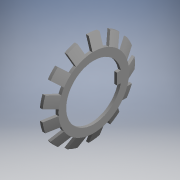
# Autodesk Inventor part: SKF_MB 5
Saved by Autodesk Inventor 2017.3 (Build 213256000, 256)
## iProperties
Part Number: SKF_MB 5
Material: Generic
Catalog Web Link: www.cadenas.de
Description: ANL_002-MB(L) lock washers
Vendor: SKF
Document SubType Name: Modeling
Designer: partserver
Manufacturer: SKF
Mass: 6 g
Surface Area: 17.574 cm^2
Volume: 0.811214 cm^3
Density: 1 g/cm^3
Appearance: PSOLRGB-175-175-175
Category: PARTsolutions
Company: SKF
Title: SKF_MB 5
Author: Cadenas PARTsolutions
Comments: MB(L) lock washers
PSOL_IDENT_0: {$CADENAS_DATA\23d-libs\skf\bearings_units_and_housings\bearing_accessories\lock_nuts\anl_002.prj},1
PSOL_IDENT_1: 59 {VTYP=3D},{NB=SKF_MB 5},{LINA=SKF_MB 5},{NN=ANL_002},{DATE=13.09.2021 11:18:37},{GEOMDATE=16.02.2
PSOL_IDENT_2: 021 08:43:28},{VERSION=},{LINEID=3400},{WBVAR=},{WBNUMERIC=}  {NB=SKF_MB 5},{LINA=SKF_MB 5},{KT=DUMM
PSOL_IDENT_3: Y},{DESIGNATION=MB 5},{DD=25.0000},{DD1=32.0000},{DD2=42.0000},{LDB=1.250},{FF=5.0000},{FM=5.000},{N
PSOL_IDENT_4: T=13},{LWM=23.0000},{MASS=0.006},{DESIGN=lockdevice_mb},{LDDD1=32},{LDDD2=42},{LDM=23},{LDFF=5},{B=0
PSOL_IDENT_5: },{LNB=0},{SS1=0},{C=0},{LWV=0},{M=23},{POPULAR=Yes}
NB: SKF_MB 5
NN: ANL_002
NT: 13
NBSYN: SKF_$DESIGNATION.
LINA: SKF_MB 5
CATALOG: SKF
DESIGNATION: MB 5
DD: 25
DD2: 42
LDB: 1.25
FM: 5
M: 23
POPULAR: Yes
SUPPLIER: SKF
ARTICLENO: SKF_MB 5
BOMINFO: SKF_MB 5
CREATOR: CADENAS GmbH
Autodesk Inventor part; units mm, degrees
ref_plane "YZ Plane" through (0, 0, 0) normal (1, 0, 0) x (0, 1, 0)
ref_plane "XZ Plane" through (0, 0, 0) normal (0, 1, 0) x (-1, 0, 0)
ref_plane "XY Plane" through (0, 0, 0) normal (0, 0, 1) x (1, 0, 0)
sketch "Sketch_1" plane through (0, 0, 0) normal (0, 0, 1) x (1, 0, 0)
  line L0 (13.75, 0) -> (-11.25, 0)
  line L1 (0, 12.5) -> (1.25, 12.5)
  line L2 (1.25, 12.5) -> (1.25, 16)
  line L3 (1.25, 16) -> (4.9805, 24)
  line L4 (4.9805, 24) -> (3.7305, 24)
  line L5 (3.7305, 24) -> (0, 16)
  line L6 (0, 16) -> (0, 12.5)
  constraints: 14 end point
revolve "Revolution1" add sketch "Sketch_1" angle 360 about axis through (13.75, 0, 0) along (1, 0, 0)
sketch "Sketch_2" plane through (0, 0, 0) normal (1, 0, 0) x (0, 1, 0)
  circle A0 centre (0, 0) radius 42
  line L0 (0.0315, 21) -> (-0.5769, 15.9896)
  arc A1 (-0.5769, 15.9896) -> (-3.2665, 15.663) centre (0, 0) ccw
  line L1 (-3.2665, 15.663) -> (-5.0562, 20.3822)
  arc A2 (-5.0562, 20.3822) -> (-9.7313, 18.6092) centre (0, 0) ccw
  line L2 (-9.7313, 18.6092) -> (-7.9415, 13.89)
  arc A3 (-7.9415, 13.89) -> (-10.1713, 12.3509) centre (0, 0) ccw
  line L3 (-10.1713, 12.3509) -> (-13.9491, 15.6978)
  arc A4 (-13.9491, 15.6978) -> (-17.2647, 11.9553) centre (0, 0) ccw
  line L4 (-17.2647, 11.9553) -> (-13.4869, 8.6084)
  arc A5 (-13.4869, 8.6084) -> (-14.746, 6.2094) centre (0, 0) ccw
  line L5 (-14.746, 6.2094) -> (-19.6465, 7.4172)
  arc A6 (-19.6465, 7.4172) -> (-20.8431, 2.5625) centre (0, 0) ccw
  line L6 (-20.8431, 2.5625) -> (-15.9425, 1.3547)
  arc A7 (-15.9425, 1.3547) -> (-15.9425, -1.3547) centre (0, 0) ccw
  line L7 (-15.9425, -1.3547) -> (-20.8431, -2.5625)
  arc A8 (-20.8431, -2.5625) -> (-19.6465, -7.4172) centre (0, 0) ccw
  line L8 (-19.6465, -7.4172) -> (-14.746, -6.2094)
  arc A9 (-14.746, -6.2094) -> (-13.4869, -8.6084) centre (0, 0) ccw
  line L9 (-13.4869, -8.6084) -> (-17.2647, -11.9553)
  arc A10 (-17.2647, -11.9553) -> (-13.9491, -15.6978) centre (0, 0) ccw
  line L10 (-13.9491, -15.6978) -> (-10.1713, -12.3509)
  arc A11 (-10.1713, -12.3509) -> (-7.9415, -13.89) centre (0, 0) ccw
  line L11 (-7.9415, -13.89) -> (-9.7313, -18.6092)
  arc A12 (-9.7313, -18.6092) -> (-5.0562, -20.3822) centre (0, 0) ccw
  line L12 (-5.0562, -20.3822) -> (-3.2665, -15.663)
  arc A13 (-3.2665, -15.663) -> (-0.5769, -15.9896) centre (0, 0) ccw
  line L13 (-0.5769, -15.9896) -> (0.0315, -21)
  arc A14 (0.0315, -21) -> (4.995, -20.3973) centre (0, 0) ccw
  line L14 (4.995, -20.3973) -> (4.3867, -15.3869)
  arc A15 (4.3867, -15.3869) -> (6.9199, -14.4262) centre (0, 0) ccw
  line L15 (6.9199, -14.4262) -> (9.7871, -18.5799)
  arc A16 (9.7871, -18.5799) -> (13.902, -15.7396) centre (0, 0) ccw
  line L16 (13.902, -15.7396) -> (11.0349, -11.5858)
  arc A17 (11.0349, -11.5858) -> (12.8315, -9.5579) centre (0, 0) ccw
  line L17 (12.8315, -9.5579) -> (17.3005, -11.9034)
  arc A18 (17.3005, -11.9034) -> (19.6241, -7.4761) centre (0, 0) ccw
  line L18 (19.6241, -7.4761) -> (15.1551, -5.1306)
  arc A19 (15.1551, -5.1306) -> (15.8035, -2.5) centre (0, 0) ccw
  line L19 (15.8035, -2.5) -> (20.8507, -2.5)
  arc A20 (20.8507, -2.5) -> (20.8507, 2.5) centre (0, 0) ccw
  line L20 (20.8507, 2.5) -> (15.8035, 2.5)
  arc A21 (15.8035, 2.5) -> (15.1551, 5.1306) centre (0, 0) ccw
  line L21 (15.1551, 5.1306) -> (19.6241, 7.4761)
  arc A22 (19.6241, 7.4761) -> (17.3005, 11.9034) centre (0, 0) ccw
  line L22 (17.3005, 11.9034) -> (12.8315, 9.5579)
  arc A23 (12.8315, 9.5579) -> (11.0349, 11.5858) centre (0, 0) ccw
  line L23 (11.0349, 11.5858) -> (13.902, 15.7396)
  arc A24 (13.902, 15.7396) -> (9.7871, 18.5799) centre (0, 0) ccw
  line L24 (9.7871, 18.5799) -> (6.9199, 14.4262)
  arc A25 (6.9199, 14.4262) -> (4.3867, 15.3869) centre (0, 0) ccw
  line L25 (4.3867, 15.3869) -> (4.995, 20.3973)
  arc A26 (4.995, 20.3973) -> (0.0315, 21) centre (0, 0) ccw
  constraints: 52 end point, 52 point on circle, 27 centre point
extrude "Extrusion1" cut sketch "Sketch_2" along normal mid plane 25
sketch "Sketch_7" plane through (0, 0, 0) normal (1, 0, 0) x (0, 0, -1)
  line L0 (-2.5, 14) -> (-2.5, 10.5)
  line L1 (-2.5, 10.5) -> (2.5, 10.5)
  line L2 (2.5, 10.5) -> (2.5, 14)
  line L3 (2.5, 14) -> (-2.5, 14)
  constraints: 8 end point
extrude "Extrusion2" add sketch "Sketch_7" along normal blind 1.25
ref_plane "mb_XY" through (-1.25, 0, 0) normal (0, 0, 1) x (1, 0, 0)
ref_plane "mb_YZ" through (-1.25, 0, 0) normal (1, 0, 0) x (0, 1, 0)
ref_plane "mb_ZX" through (-1.25, 0, 0) normal (0, 1, 0) x (0, 0, 1)
ref_plane "mb2_XY" through (0, 0, 0) normal (0, 0, 1) x (1, 0, 0)
ref_plane "mb2_YZ" through (0, 0, 0) normal (1, 0, 0) x (0, 1, 0)
ref_plane "mb2_ZX" through (0, 0, 0) normal (0, 1, 0) x (0, 0, 1)
ref_plane "to_locknut_XY" through (1.25, 0, 0) normal (1, 0, 0) x (0, 0, -1)
ref_plane "to_locknut_YZ" through (1.25, 0, 0) normal (0, 0, -1) x (0, 1, 0)
ref_plane "to_locknut_ZX" through (1.25, 0, 0) normal (0, 1, 0) x (1, 0, 0)
body "Solid1"
